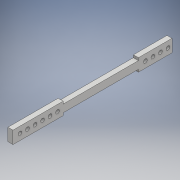
# Autodesk Inventor part: Jumper
Saved by Autodesk Inventor 2018 (Build 220112000, 112)
## iProperties
Created: 2019-04-03
Part Number: Jumper
Material: Типовые
Document SubType Name: Modeling
Designer: cosko
Density: 1 g/cm^3
Appearance: По умолчанию
Author: cosko
Autodesk Inventor part; units mm, degrees
ref_plane "YZ Plane" through (0, 0, 0) normal (1, 0, 0) x (0, 1, 0)
ref_plane "XY Plane" through (0, 0, 0) normal (0, 0, 1) x (1, 0, 0)
sketch "Эскиз1" plane through (0, 0, 0) normal (0, 0, 1) x (1, 0, 0)
  circle A0 centre (0, 0) radius 2.5
  circle A1 centre (0, 0) radius 10
  dimension "d0" = 5
  dimension "d1" = 20
  constraints: 2 centre point, 2 coincident
  measures "d0" diameter of A0
  measures "d1" diameter of A1
extrude "Выдавливание1" add sketch "Эскиз1" along normal blind 5
ref_plane "РабПлоскость1" through (0, 11, 0) normal (0, 1, 0) x (-1, 0, 0)
sketch "Эскиз2" plane through (0, 11, 0) normal (0, 1, 0) x (-1, 0, 0)
  line L0 (2.5, 0) -> (2.5, 5) projected
  line L1 (10, 5) -> (-10, 5) projected
  line L2 (-10, 0) -> (10, 0) projected
  circle A0 centre (0, 2.5) radius 1.5
  point P0 (0, 0)
  dimension "d5" = 3
  constraints: 1 centre point
  measures "d5" diameter of A0
extrude "Выдавливание2" cut sketch "Эскиз2" against normal blind 10
sketch "Эскиз3" plane through (0, 0, 5) normal (0, 0, 1) x (1, 0, 0)
  circle A0 centre (0, 0) radius 2.5 construction
  line L0 (0, 2.5) -> (0, 10) construction
  circle A1 centre (0, 0) radius 10 construction
  circle A2 centre (0, 6.25) radius 1.5
  circle A3 centre (-6.25, 0) radius 1.5
  circle A4 centre (0, -6.25) radius 1.5
  circle A5 centre (6.25, 0) radius 1.5
  dimension "d8" = 3
  dimension "d11" = 360
  constraints: 4 centre point, 2 end point, 2 vertical alignment, 1 midpoint, 1 vertical, 11 other
  measures "d8" diameter of A2
extrude "Выдавливание3" cut sketch "Эскиз3" against normal blind 6
sketch "Эскиз4" plane through (0, 0, 5) normal (0, 0, 1) x (1, 0, 0)
  circle A0 centre (0, -6.25) radius 1.5 projected
  circle A1 centre (0, 6.25) radius 1.5 projected
  circle A2 centre (-6.25, 0) radius 1.5 projected
  circle A3 centre (6.25, 0) radius 1.5 projected
  circle A4 centre (0, 0) radius 2.5 projected
  circle A5 centre (0, 0) radius 10 projected
  circle A6 centre (0, 0) radius 10 projected
  line L0 (-8.7999, 4.75) -> (8.7999, 4.75)
  arc A7 (-8.7999, 4.75) -> (8.7999, 4.75) centre (0, 0) ccw
  circle A8 centre (0, 0) radius 2.5 projected
  circle A9 centre (-6.25, 0) radius 1.5 projected
  circle A10 centre (6.25, 0) radius 1.5 projected
  circle A11 centre (0, -6.25) radius 1.5 projected
  constraints: 4 point on circle, 2 end point, 1 centre point, 1 coincident, 1 concentric, 1 horizontal
extrude "Выдавливание4" add sketch "Эскиз4" along normal blind 6 separate body contours L0 A5 picked at (4.8814, -4.6474)
sketch "Эскиз5" plane through (0, 0, 11) normal (0, 0, 1) x (1, 0, 0)
  circle A0 centre (0, 0) radius 2.5 projected
  circle A1 centre (6.25, 0) radius 1.5 projected
  circle A2 centre (-6.25, 0) radius 1.5 projected
  circle A3 centre (0, -6.25) radius 1.5 projected
  arc A4 (-8.7999, 4.75) -> (8.7999, 4.75) centre (0, 0) ccw projected
  line L0 (8.7999, 4.75) -> (-8.7999, 4.75) projected
  circle A5 centre (-6.25, 0) radius 1.5 projected
  circle A6 centre (6.25, 0) radius 1.5 projected
  line L1 (4.75, 0) -> (4.75, -60)
  line L2 (4.75, -60) -> (-4.75, -60)
  line L3 (-4.75, -60) -> (-4.75, 0)
  line L4 (-4.75, 0) -> (-2.5, 0)
  line L5 (2.5, 0) -> (4.75, 0)
  dimension "d17" = 60
  constraints: 10 end point, 3 parallel, 2 horizontal, 2 horizontal alignment, 2 perpendicular, 2 point on circle, 2 other
  measures "d17" distance of L1.start L1.end
extrude "Выдавливание5" add sketch "Эскиз5" against normal blind 6 contours L5 L1 A4 L3 L4 A0 | L1 L2 L3 A4 bodies 2
sketch "Эскиз6" plane through (4.75, -60, 11) normal (1, 0, 0) x (0, 0, -1)
  line L0 (-2, -20) -> (-2, 20)
  line L1 (-2, 20) -> (8, 20)
  line L2 (8, 20) -> (8, -20)
  line L3 (8, -20) -> (-2, -20)
  line L4 (0, 0) -> (6, 0) projected
  line L5 (-2, -20) -> (8, 20) construction
  line L6 (-2, 20) -> (8, -20) construction
  point P0 (11, 60)
  point P1 (3, 0)
  dimension "d20" = 40
  dimension "d21" = 10
  constraints: 12 end point, 3 midpoint, 2 parallel, 1 perpendicular, 1 vertical
  measures "d20" distance of L0.start L0.end
  measures "d21" distance of L0.end L1.end
extrude "Выдавливание6" add sketch "Эскиз6" against normal up to surface (9.5 mm away) bodies 2
sketch "Эскиз7" plane through (4.75, -8.7999, 11) normal (1, 0, 0) x (0, 0, -1)
  line L0 (-2, -31.2001) -> (0, -31.2001) projected
  line L1 (-2, -71.2001) -> (-2, -31.2001) projected
  line L2 (8, -71.2001) -> (-2, -71.2001) projected
  line L3 (8, -31.2001) -> (8, -71.2001) projected
  line L4 (6, -31.2001) -> (8, -31.2001) projected
  line L5 (6, 0) -> (6, -31.2001) projected
  line L6 (0, 0) -> (6, 0) projected
  line L7 (0, -31.2001) -> (0, 0) projected
  line L8 (-2, -31.2001) -> (8, -31.2001) construction
  line L9 (3, -31.2001) -> (3, -71.2001) construction
  line L10 (8, -31.2001) -> (8, -71.2001) construction
  line L11 (8, -51.2001) -> (-2, -51.2001) construction
  line L12 (-2, -71.2001) -> (-2, -31.2001) construction
  line L13 (3, -31.2001) -> (3, -34.2001) construction
  line L14 (3, -34.2001) -> (3, -37.2001) construction
  circle A0 centre (3, -35.7001) radius 1.5
  circle A1 centre (3, -41.7001) radius 1.5
  circle A2 centre (3, -47.7001) radius 1.5
  circle A3 centre (3, -53.7001) radius 1.5
  circle A4 centre (3, -59.7001) radius 1.5
  circle A5 centre (3, -65.7001) radius 1.5
  point P0 (11, 8.7999)
  point P1 (3, -40.2001)
  point P2 (3, -46.2001)
  point P3 (3, -52.2001)
  point P4 (3, -58.2001)
  point P5 (3, -64.2001)
  dimension "d24" = 3
  dimension "d25" = 3
  dimension "d28" = 6
  constraints: 10 end point, 6 vertical, 6 vertical alignment, 5 midpoint, 2 point on line, 1 horizontal, 22 other
  measures "d24" distance of L9.start L13.end
  measures "d25" distance of L13.end L14.end
  measures "d28" distance of point (3, -35.7) point (3, -41.7)
extrude "Выдавливание7" cut sketch "Эскиз7" against normal blind 10 contours A0 | A1 | A2 | A3 | A4 | A5 bodies 2
sketch "Эскиз8" plane through (4.75, -8.7999, 11) normal (1, 0, 0) x (0, 0, -1)
  line L0 (-2, -71.2001) -> (-2, -31.2001) projected
  line L1 (8, -71.2001) -> (-2, -71.2001)
  line L2 (-2, -71.2001) -> (-2, -44.4041)
  line L3 (-2, -44.4041) -> (8, -44.4041)
  line L4 (8, -44.4041) -> (8, -71.2001)
  circle A0 centre (3, -47.7001) radius 1.5 projected
  circle A1 centre (3, -53.7001) radius 1.5 projected
  circle A2 centre (3, -59.7001) radius 1.5 projected
  circle A3 centre (3, -65.7001) radius 1.5 projected
  point P0 (11, 8.7999)
  constraints: 8 end point, 2 parallel, 1 horizontal, 1 perpendicular, 1 point on line
extrude "Выдавливание8" add sketch "Эскиз8" along normal blind 4 separate body
sketch "Эскиз9" plane through (8.75, -8.7999, 11) normal (1, 0, 0) x (0, 0, -1)
  circle A0 centre (3, -65.7001) radius 1.5 projected
  circle A1 centre (3, -59.7001) radius 1.5 projected
  circle A2 centre (3, -53.7001) radius 1.5 projected
  circle A3 centre (3, -47.7001) radius 1.5 projected
  line L0 (-2, -71.2001) -> (8, -71.2001) projected
  line L1 (8, -71.2001) -> (8, -44.4041) projected
  line L2 (8, -44.4041) -> (-2, -44.4041) projected
  line L3 (-2, -44.4041) -> (-2, -71.2001) projected
  line L4 (-2, -31.2001) -> (0, -31.2001) construction
  line L5 (0, -31.2001) -> (6, -31.2001) construction
  line L6 (6, -31.2001) -> (6, -71.2001) construction
  line L7 (6, -71.2001) -> (0, -71.2001) construction
  line L8 (0, -71.2001) -> (0, -31.2001) construction
  line L9 (0, -71.2001) -> (6, -71.2001)
  line L10 (6, -71.2001) -> (6, -171.2001)
  line L11 (6, -171.2001) -> (0, -171.2001)
  line L12 (0, -171.2001) -> (0, -71.2001)
  line L13 (8, -71.2001) -> (-2, -71.2001) projected
  point P0 (11, 8.7999)
  dimension "d37" = 6
  dimension "d38" = 100
  constraints: 16 end point, 4 parallel, 2 perpendicular, 1 collinear, 1 horizontal, 1 point on line
  measures "d37" distance of L6.end L7.end
  measures "d38" distance of L6.end L10.end
extrude "Выдавливание9" add sketch "Эскиз9" against normal blind 4 contours L0 L10 L11 L12 bodies 3
sketch "Эскиз10" plane through (8.75, -8.7999, 11) normal (1, 0, 0) x (0, 0, -1)
  line L0 (-2, -31.2001) -> (0, -31.2001) projected
  line L1 (8, -31.2001) -> (6, -31.2001) projected
  line L2 (-2, -31.2001) -> (8, -31.2001)
  line L3 (8, -131.2001) -> (8, -171.2001)
  line L4 (8, -171.2001) -> (-2, -171.2001)
  line L5 (-2, -171.2001) -> (-2, -131.2001)
  line L6 (8, -171.2001) -> (-2, -171.2001)
  line L7 (-2, -171.2001) -> (-2, -131.2001)
  line L8 (-2, -131.2001) -> (8, -131.2001)
  line L9 (8, -131.2001) -> (8, -171.2001)
  line L10 (3, -131.2001) -> (3, -134.2001) construction
  line L11 (3, -134.2001) -> (3, -137.2001) construction
  circle A0 centre (3, -135.7001) radius 1.5
  circle A1 centre (3, -141.7001) radius 1.5
  circle A2 centre (3, -147.7001) radius 1.5
  circle A3 centre (3, -153.7001) radius 1.5
  circle A4 centre (3, -159.7001) radius 1.5
  circle A5 centre (3, -165.7001) radius 1.5
  point P0 (11, 8.7999)
  point P1 (3, -140.2001)
  point P2 (3, -146.2001)
  point P3 (3, -152.2001)
  point P4 (3, -158.2001)
  point P5 (3, -164.2001)
  dimension "d41" = 140
  dimension "d42" = 40
  dimension "d43" = 3
  dimension "d44" = 3
  dimension "d47" = 6
  constraints: 20 end point, 7 vertical, 6 vertical alignment, 4 parallel, 2 horizontal, 2 midpoint, 2 perpendicular, 1 point on line, 22 other
  measures "d41" distance of L1.start L3.end
  measures "d42" distance of L5.end L6.end
  measures "d43" distance of L10.start L10.end
  measures "d44" distance of L10.end L11.end
  measures "d47" distance of point (3, -135.7) point (3, -141.7)
extrude "Выдавливание10" add sketch "Эскиз10" against normal blind 4 bodies 3
extrude "Выдавливание11" cut sketch "Эскиз10" against normal blind 4 contours A0 | A1 | A2 | A3 | A4 | A5 bodies 3
sketch "Эскиз11" plane through (4.75, -8.7999, 11) normal (1, 0, 0) x (0, 0, -1)
  circle A0 centre (3, -59.7001) radius 1.5 projected
  circle A1 centre (3, -47.7001) radius 1.5 projected
  circle A2 centre (3, -35.7001) radius 1.5 projected
  circle A3 centre (3, -41.7001) radius 1.5 projected
  circle A4 centre (3, -53.7001) radius 1.5 projected
  circle A5 centre (3, -65.7001) radius 1.5 projected
  line L0 (-2, -31.2001) -> (0, -31.2001) projected
  line L1 (-2, -71.2001) -> (-2, -31.2001) projected
  line L2 (8, -71.2001) -> (-2, -71.2001) projected
  line L3 (8, -31.2001) -> (8, -71.2001) projected
  line L4 (6, -31.2001) -> (8, -31.2001) projected
  line L5 (6, 0) -> (6, -31.2001) projected
  line L6 (0, 0) -> (6, 0) projected
  line L7 (0, -31.2001) -> (0, 0) projected
  line L8 (0, 0) -> (0, -31.2001) projected
  line L9 (0, -31.2001) -> (6, -31.2001)
  point P0 (11, 8.7999)
  constraints: 2 end point, 1 perpendicular
extrude "Выдавливание12" cut sketch "Эскиз11" against normal blind 3 contours L0 L9 L4 L3 L2 L1 bodies 2
sketch "Эскиз12" plane through (0, 0, 5) normal (0, 0, -1) x (-1, 0, 0)
  line L0 (-4.75, -40) -> (-1.75, -40) projected
  line L1 (-1.75, -40) -> (-4.75, -37)
  line L2 (-4.75, -40) -> (-4.75, -8.7999) projected
  line L3 (-1.75, -40) -> (2.4926, -40) construction
  line L4 (-4.75, -40) -> (-4.75, -37)
  point P0 (0, 0)
  dimension "d58" = 135
  constraints: 6 end point, 1 collinear, 1 equal length, 1 horizontal, 1 point on line
  measures "d58" angle of L3 L1
extrude "Выдавливание13" cut sketch "Эскиз12" against normal blind 6 bodies 2
